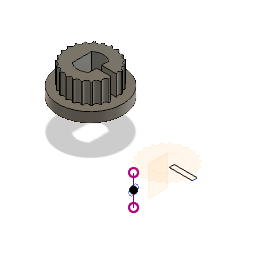
fully-gear v4 (Autodesk Fusion 360 design; units mm, degrees)
Autodesk Fusion 360 part; units mm, degrees
sketch "Sketch1" plane through (0, 0, 0) normal (0, 1, 0) x (1, 0, 0)
  arc A0 (-0.5173, 4.9732) -> (0.5937, 4.9646) centre (0.04, 5.1956) ccw
  arc A1 (-1.8399, 4.6492) -> (-0.7677, 4.9407) centre (-1.3633, 5.0137) ccw
  arc A2 (-3.026, 3.9804) -> (-2.0722, 4.5504) centre (-2.6654, 4.46) ccw
  arc A3 (-3.9877, 3.0164) -> (-3.2231, 3.8225) centre (-3.7698, 3.5755) ccw
  arc A4 (-4.6536, 1.8287) -> (-4.1349, 2.8112) centre (-4.5947, 2.4258) ccw
  arc A5 (-4.9744, 0.5053) -> (-4.74, 1.5914) centre (-5.0788, 1.0962) ccw
  arc A6 (-4.9263, -0.8555) -> (-4.9936, 0.2535) centre (-5.1862, -0.3147) ccw
  arc A7 (-4.5128, -2.1528) -> (-4.8768, -1.1031) centre (-4.909, -1.7022) ccw
  arc A8 (-3.7646, -3.2905) -> (-4.3983, -2.3779) centre (-4.2677, -2.9635) ccw
  arc A9 (-2.7372, -4.1842) -> (-3.5937, -3.4764) centre (-3.3099, -4.005) ccw
  arc A10 (-1.5068, -4.7675) -> (-2.5225, -4.3171) centre (-2.1066, -4.7495) ccw
  arc A11 (-0.1647, -4.9973) -> (-1.2642, -4.8375) centre (-0.7471, -5.1417) ccw
  arc A12 (1.1897, -4.8564) -> (0.0878, -4.9992) centre (0.6679, -5.1526) ccw
  arc A13 (2.4558, -4.3554) -> (1.4333, -4.7902) centre (2.0333, -4.7814) ccw
  arc A14 (3.5398, -3.5313) -> (2.6726, -4.2258) centre (3.2479, -4.0555) ccw
  arc A15 (4.3612, -2.4453) -> (3.7136, -3.3481) centre (4.2216, -3.0288) ccw
  arc A16 (4.8593, -1.178) -> (4.4791, -2.222) centre (4.8822, -1.7775) ccw
  arc A17 (4.9969, 0.1767) -> (4.9125, -0.9311) centre (5.1807, -0.3944) ccw
  arc A18 (4.7639, 1.5183) -> (4.9816, 0.4288) centre (5.095, 1.0179) ccw
  arc A19 (4.1776, 2.7473) -> (4.6812, 1.7569) centre (4.6315, 2.3548) ccw
  arc A20 (3.2815, 3.7725) -> (4.0336, 2.9547) centre (3.8244, 3.5171) ccw
  arc A21 (2.142, 4.518) -> (3.0868, 3.9334) centre (2.7337, 4.4184) ccw
  arc A22 (0.8436, 4.9283) -> (1.9112, 4.6203) centre (1.4402, 4.9921) ccw
  arc A23 (4.1776, 2.7473) -> (4.0336, 2.9547) centre (0, 0) ccw
  arc A24 (4.7639, 1.5183) -> (4.6812, 1.7569) centre (0, 0) ccw
  arc A25 (3.2815, 3.7725) -> (3.0868, 3.9334) centre (0, 0) ccw
  arc A26 (2.142, 4.518) -> (1.9112, 4.6203) centre (0, 0) ccw
  arc A27 (0.8436, 4.9283) -> (0.5937, 4.9646) centre (0, 0) ccw
  arc A28 (-0.5173, 4.9732) -> (-0.7677, 4.9407) centre (0, 0) ccw
  arc A29 (-1.8399, 4.6492) -> (-2.0722, 4.5504) centre (0, 0) ccw
  arc A30 (-3.026, 3.9804) -> (-3.2231, 3.8225) centre (0, 0) ccw
  arc A31 (-3.9877, 3.0164) -> (-4.1349, 2.8112) centre (0, 0) ccw
  arc A32 (-4.6536, 1.8287) -> (-4.74, 1.5914) centre (0, 0) ccw
  arc A33 (-4.9744, 0.5053) -> (-4.9936, 0.2535) centre (0, 0) ccw
  arc A34 (-4.9263, -0.8555) -> (-4.8768, -1.1031) centre (0, 0) ccw
  arc A35 (-4.5128, -2.1528) -> (-4.3983, -2.3779) centre (0, 0) ccw
  arc A36 (-3.7646, -3.2905) -> (-3.5937, -3.4764) centre (0, 0) ccw
  arc A37 (-2.7372, -4.1842) -> (-2.5225, -4.3171) centre (0, 0) ccw
  arc A38 (-1.5068, -4.7675) -> (-1.2642, -4.8375) centre (0, 0) ccw
  arc A39 (-0.1647, -4.9973) -> (0.0878, -4.9992) centre (0, 0) ccw
  arc A40 (1.1897, -4.8564) -> (1.4333, -4.7902) centre (0, 0) ccw
  arc A41 (2.4558, -4.3554) -> (2.6726, -4.2258) centre (0, 0) ccw
  arc A42 (3.5398, -3.5313) -> (3.7136, -3.3481) centre (0, 0) ccw
  arc A43 (4.3612, -2.4453) -> (4.4791, -2.222) centre (0, 0) ccw
  arc A44 (4.8593, -1.178) -> (4.9125, -0.9311) centre (0, 0) ccw
  arc A45 (4.9969, 0.1767) -> (4.9816, 0.4288) centre (0, 0) ccw
  dimension "d1" = 10
  dimension "d2" = 0.6
  dimension "d4" = 360
  measures "d1" diameter of A25
  measures "d2" radius of A0
sketch "Sketch2" plane through (0.0017, 0, 0.0141) normal (0, 1, 0) x (1, 0, 0)
  line L0 (1.7, 1.9007) -> (1.7, -1.9672)
  line L1 (-1.7017, -1.9658) -> (-1.7017, 1.8992)
  arc A0 (-1.7017, -1.9658) -> (1.7, -1.9672) centre (0, 0) ccw
  arc A1 (1.7, 1.9007) -> (-1.7017, 1.8992) centre (0, 0) ccw
  dimension "d5" = 5.2
  dimension "d7" = 1.7
  dimension "d12" = 1.7
  measures "d5" diameter of A0
  measures "d7" distance of L1
  measures "d12" distance of L0 A0.centre
extrude "Extrude1" add sketch "Sketch1" along normal blind 6.1 makes body 1
extrude "Extrude2" cut sketch "Sketch2" along normal blind 12.5 bodies 1
sketch "Sketch3" plane through (-1.7, 0, 0) normal (1, 0, 0) x (0, 0, -1)
  line L0 (1.885, 6.1) -> (-1.9799, 6.1)
  line L1 (-1.9799, 6.1) -> (-1.9799, 0)
  line L2 (-1.9799, 0) -> (1.885, 0)
  line L3 (1.885, 0) -> (1.885, 6.1)
  circle A0 centre (-4.9992, 3.05) radius 0.947
  line L4 (-4.9992, 0) -> (-4.9992, 6.1)
sketch "Sketch4" plane through (0, 6.1, 0) normal (0, 1, 0) x (-1, 0, 0)
  line L0 (1.7, 1.9799) -> (1.7, -1.885)
  arc A0 (-1.7017, -1.8865) -> (1.7, -1.885) centre (-0.0017, 0.0141) ccw
  line L1 (-1.7017, -1.8865) -> (-1.7017, 1.9814)
  arc A1 (1.7, 1.9799) -> (-1.7017, 1.9814) centre (-0.0017, 0.0141) ccw
  arc A2 (-4.8593, 1.178) -> (-4.9125, 0.9311) centre (0, 0) ccw
  arc A3 (-4.9969, -0.1767) -> (-4.9125, 0.9311) centre (-5.1807, 0.3944) ccw
  arc A4 (-4.9969, -0.1767) -> (-4.9816, -0.4288) centre (0, 0) ccw
  arc A5 (-4.7639, -1.5183) -> (-4.9816, -0.4288) centre (-5.095, -1.0179) ccw
  arc A6 (-4.7639, -1.5183) -> (-4.6812, -1.7569) centre (0, 0) ccw
  arc A7 (-4.1776, -2.7473) -> (-4.6812, -1.7569) centre (-4.6315, -2.3548) ccw
  arc A8 (-4.1776, -2.7473) -> (-4.0336, -2.9547) centre (0, 0) ccw
  arc A9 (-3.2815, -3.7725) -> (-4.0336, -2.9547) centre (-3.8244, -3.5171) ccw
  arc A10 (-3.2815, -3.7725) -> (-3.0868, -3.9334) centre (0, 0) ccw
  arc A11 (-2.142, -4.518) -> (-3.0868, -3.9334) centre (-2.7337, -4.4184) ccw
  arc A12 (-2.142, -4.518) -> (-1.9112, -4.6203) centre (0, 0) ccw
  arc A13 (-0.8436, -4.9283) -> (-1.9112, -4.6203) centre (-1.4402, -4.9921) ccw
  arc A14 (-0.8436, -4.9283) -> (-0.5937, -4.9646) centre (0, 0) ccw
  arc A15 (0.5173, -4.9732) -> (-0.5937, -4.9646) centre (-0.04, -5.1956) ccw
  arc A16 (0.5173, -4.9732) -> (0.7677, -4.9407) centre (0, 0) ccw
  arc A17 (1.8399, -4.6492) -> (0.7677, -4.9407) centre (1.3633, -5.0137) ccw
  arc A18 (1.8399, -4.6492) -> (2.0722, -4.5504) centre (0, 0) ccw
  arc A19 (3.026, -3.9804) -> (2.0722, -4.5504) centre (2.6654, -4.46) ccw
  arc A20 (3.026, -3.9804) -> (3.2231, -3.8225) centre (0, 0) ccw
  arc A21 (3.9877, -3.0164) -> (3.2231, -3.8225) centre (3.7698, -3.5755) ccw
  arc A22 (3.9877, -3.0164) -> (4.1349, -2.8112) centre (0, 0) ccw
  arc A23 (4.6536, -1.8287) -> (4.1349, -2.8112) centre (4.5947, -2.4258) ccw
  arc A24 (4.6536, -1.8287) -> (4.74, -1.5914) centre (0, 0) ccw
  arc A25 (4.9744, -0.5053) -> (4.74, -1.5914) centre (5.0788, -1.0962) ccw
  arc A26 (4.9744, -0.5053) -> (4.9936, -0.2535) centre (0, 0) ccw
  arc A27 (4.9263, 0.8555) -> (4.9936, -0.2535) centre (5.1862, 0.3147) ccw
  arc A28 (4.9263, 0.8555) -> (4.8768, 1.1031) centre (0, 0) ccw
  arc A29 (4.5128, 2.1528) -> (4.8768, 1.1031) centre (4.909, 1.7022) ccw
  arc A30 (4.5128, 2.1528) -> (4.3983, 2.3779) centre (0, 0) ccw
  arc A31 (3.7646, 3.2905) -> (4.3983, 2.3779) centre (4.2677, 2.9635) ccw
  arc A32 (3.7646, 3.2905) -> (3.5937, 3.4764) centre (0, 0) ccw
  arc A33 (2.7372, 4.1842) -> (3.5937, 3.4764) centre (3.3099, 4.005) ccw
  arc A34 (2.7372, 4.1842) -> (2.5225, 4.3171) centre (0, 0) ccw
  arc A35 (1.5068, 4.7675) -> (2.5225, 4.3171) centre (2.1066, 4.7495) ccw
  arc A36 (1.5068, 4.7675) -> (1.2642, 4.8375) centre (0, 0) ccw
  arc A37 (0.1647, 4.9973) -> (1.2642, 4.8375) centre (0.7471, 5.1417) ccw
  arc A38 (0.1647, 4.9973) -> (-0.0878, 4.9992) centre (0, 0) ccw
  arc A39 (-1.1897, 4.8564) -> (-0.0878, 4.9992) centre (-0.6679, 5.1526) ccw
  arc A40 (-1.1897, 4.8564) -> (-1.4333, 4.7902) centre (0, 0) ccw
  arc A41 (-2.4558, 4.3554) -> (-1.4333, 4.7902) centre (-2.0333, 4.7814) ccw
  arc A42 (-2.4558, 4.3554) -> (-2.6726, 4.2258) centre (0, 0) ccw
  arc A43 (-3.5398, 3.5313) -> (-2.6726, 4.2258) centre (-3.2479, 4.0555) ccw
  arc A44 (-3.5398, 3.5313) -> (-3.7136, 3.3481) centre (0, 0) ccw
  arc A45 (-4.3612, 2.4453) -> (-3.7136, 3.3481) centre (-4.2216, 3.0288) ccw
  arc A46 (-4.3612, 2.4453) -> (-4.4791, 2.222) centre (0, 0) ccw
  arc A47 (-4.8593, 1.178) -> (-4.4791, 2.222) centre (-4.8822, 1.7775) ccw
ref_plane "WorkPlane2" through (0, 3.1, 0) normal (0, 1, 0) x (-1, 0, 0)
sketch "Sketch6" plane through (0, 6.1, 0) normal (0, 1, 0) x (-1, 0, 0)
  line L0 (1.7, 1.9799) -> (1.7, -1.885)
  arc A0 (-1.7017, -1.8865) -> (1.7, -1.885) centre (-0.0017, 0.0141) ccw
  line L1 (-1.7017, -1.8865) -> (-1.7017, 1.9814)
  arc A1 (1.7, 1.9799) -> (-1.7017, 1.9814) centre (-0.0017, 0.0141) ccw
  arc A2 (-4.8593, 1.178) -> (-4.9125, 0.9311) centre (0, 0) ccw
  arc A3 (-4.9969, -0.1767) -> (-4.9125, 0.9311) centre (-5.1807, 0.3944) ccw
  arc A4 (-4.9969, -0.1767) -> (-4.9816, -0.4288) centre (0, 0) ccw
  arc A5 (-4.7639, -1.5183) -> (-4.9816, -0.4288) centre (-5.095, -1.0179) ccw
  arc A6 (-4.7639, -1.5183) -> (-4.6812, -1.7569) centre (0, 0) ccw
  arc A7 (-4.1776, -2.7473) -> (-4.6812, -1.7569) centre (-4.6315, -2.3548) ccw
  arc A8 (-4.1776, -2.7473) -> (-4.0336, -2.9547) centre (0, 0) ccw
  arc A9 (-3.2815, -3.7725) -> (-4.0336, -2.9547) centre (-3.8244, -3.5171) ccw
  arc A10 (-3.2815, -3.7725) -> (-3.0868, -3.9334) centre (0, 0) ccw
  arc A11 (-2.142, -4.518) -> (-3.0868, -3.9334) centre (-2.7337, -4.4184) ccw
  arc A12 (-2.142, -4.518) -> (-1.9112, -4.6203) centre (0, 0) ccw
  arc A13 (-0.8436, -4.9283) -> (-1.9112, -4.6203) centre (-1.4402, -4.9921) ccw
  arc A14 (-0.8436, -4.9283) -> (-0.5937, -4.9646) centre (0, 0) ccw
  arc A15 (0.5173, -4.9732) -> (-0.5937, -4.9646) centre (-0.04, -5.1956) ccw
  arc A16 (0.5173, -4.9732) -> (0.7677, -4.9407) centre (0, 0) ccw
  arc A17 (1.8399, -4.6492) -> (0.7677, -4.9407) centre (1.3633, -5.0137) ccw
  arc A18 (1.8399, -4.6492) -> (2.0722, -4.5504) centre (0, 0) ccw
  arc A19 (3.026, -3.9804) -> (2.0722, -4.5504) centre (2.6654, -4.46) ccw
  arc A20 (3.026, -3.9804) -> (3.2231, -3.8225) centre (0, 0) ccw
  arc A21 (3.9877, -3.0164) -> (3.2231, -3.8225) centre (3.7698, -3.5755) ccw
  arc A22 (3.9877, -3.0164) -> (4.1349, -2.8112) centre (0, 0) ccw
  arc A23 (4.6536, -1.8287) -> (4.1349, -2.8112) centre (4.5947, -2.4258) ccw
  arc A24 (4.6536, -1.8287) -> (4.74, -1.5914) centre (0, 0) ccw
  arc A25 (4.9744, -0.5053) -> (4.74, -1.5914) centre (5.0788, -1.0962) ccw
  arc A26 (4.9744, -0.5053) -> (4.9936, -0.2535) centre (0, 0) ccw
  arc A27 (4.9263, 0.8555) -> (4.9936, -0.2535) centre (5.1862, 0.3147) ccw
  arc A28 (4.9263, 0.8555) -> (4.8768, 1.1031) centre (0, 0) ccw
  arc A29 (4.5128, 2.1528) -> (4.8768, 1.1031) centre (4.909, 1.7022) ccw
  arc A30 (4.5128, 2.1528) -> (4.3983, 2.3779) centre (0, 0) ccw
  arc A31 (3.7646, 3.2905) -> (4.3983, 2.3779) centre (4.2677, 2.9635) ccw
  arc A32 (3.7646, 3.2905) -> (3.5937, 3.4764) centre (0, 0) ccw
  arc A33 (2.7372, 4.1842) -> (3.5937, 3.4764) centre (3.3099, 4.005) ccw
  arc A34 (2.7372, 4.1842) -> (2.5225, 4.3171) centre (0, 0) ccw
  arc A35 (1.5068, 4.7675) -> (2.5225, 4.3171) centre (2.1066, 4.7495) ccw
  arc A36 (1.5068, 4.7675) -> (1.2642, 4.8375) centre (0, 0) ccw
  arc A37 (0.1647, 4.9973) -> (1.2642, 4.8375) centre (0.7471, 5.1417) ccw
  arc A38 (0.1647, 4.9973) -> (-0.0878, 4.9992) centre (0, 0) ccw
  arc A39 (-1.1897, 4.8564) -> (-0.0878, 4.9992) centre (-0.6679, 5.1526) ccw
  arc A40 (-1.1897, 4.8564) -> (-1.4333, 4.7902) centre (0, 0) ccw
  arc A41 (-2.4558, 4.3554) -> (-1.4333, 4.7902) centre (-2.0333, 4.7814) ccw
  arc A42 (-2.4558, 4.3554) -> (-2.6726, 4.2258) centre (0, 0) ccw
  arc A43 (-3.5398, 3.5313) -> (-2.6726, 4.2258) centre (-3.2479, 4.0555) ccw
  arc A44 (-3.5398, 3.5313) -> (-3.7136, 3.3481) centre (0, 0) ccw
  arc A45 (-4.3612, 2.4453) -> (-3.7136, 3.3481) centre (-4.2216, 3.0288) ccw
  arc A46 (-4.3612, 2.4453) -> (-4.4791, 2.222) centre (0, 0) ccw
  arc A47 (-4.8593, 1.178) -> (-4.4791, 2.222) centre (-4.8822, 1.7775) ccw
  circle A48 centre (0, 0) radius 6
  dimension "d25" = 12
  measures "d25" diameter of A48
sketch "Sketch8" plane through (0, 6.1, 0) normal (0, 1, 0) x (-1, 0, 0)
  line L0 (1.7, 1.9799) -> (1.7, -1.885)
  arc A0 (-1.7017, -1.8865) -> (1.7, -1.885) centre (-0.0017, 0.0141) ccw
  line L1 (-1.7017, -1.8865) -> (-1.7017, 1.9814)
  arc A1 (1.7, 1.9799) -> (-1.7017, 1.9814) centre (-0.0017, 0.0141) ccw
  arc A2 (-4.8593, 1.178) -> (-4.9125, 0.9311) centre (0, 0) ccw
  arc A3 (-4.9969, -0.1767) -> (-4.9125, 0.9311) centre (-5.1807, 0.3944) ccw
  arc A4 (-4.9969, -0.1767) -> (-4.9816, -0.4288) centre (0, 0) ccw
  arc A5 (-4.7639, -1.5183) -> (-4.9816, -0.4288) centre (-5.095, -1.0179) ccw
  arc A6 (-4.7639, -1.5183) -> (-4.6812, -1.7569) centre (0, 0) ccw
  arc A7 (-4.1776, -2.7473) -> (-4.6812, -1.7569) centre (-4.6315, -2.3548) ccw
  arc A8 (-4.1776, -2.7473) -> (-4.0336, -2.9547) centre (0, 0) ccw
  arc A9 (-3.2815, -3.7725) -> (-4.0336, -2.9547) centre (-3.8244, -3.5171) ccw
  arc A10 (-3.2815, -3.7725) -> (-3.0868, -3.9334) centre (0, 0) ccw
  arc A11 (-2.142, -4.518) -> (-3.0868, -3.9334) centre (-2.7337, -4.4184) ccw
  arc A12 (-2.142, -4.518) -> (-1.9112, -4.6203) centre (0, 0) ccw
  arc A13 (-0.8436, -4.9283) -> (-1.9112, -4.6203) centre (-1.4402, -4.9921) ccw
  arc A14 (-0.8436, -4.9283) -> (-0.5937, -4.9646) centre (0, 0) ccw
  arc A15 (0.5173, -4.9732) -> (-0.5937, -4.9646) centre (-0.04, -5.1956) ccw
  arc A16 (0.5173, -4.9732) -> (0.7677, -4.9407) centre (0, 0) ccw
  arc A17 (1.8399, -4.6492) -> (0.7677, -4.9407) centre (1.3633, -5.0137) ccw
  arc A18 (1.8399, -4.6492) -> (2.0722, -4.5504) centre (0, 0) ccw
  arc A19 (3.026, -3.9804) -> (2.0722, -4.5504) centre (2.6654, -4.46) ccw
  arc A20 (3.026, -3.9804) -> (3.2231, -3.8225) centre (0, 0) ccw
  arc A21 (3.9877, -3.0164) -> (3.2231, -3.8225) centre (3.7698, -3.5755) ccw
  arc A22 (3.9877, -3.0164) -> (4.1349, -2.8112) centre (0, 0) ccw
  arc A23 (4.6536, -1.8287) -> (4.1349, -2.8112) centre (4.5947, -2.4258) ccw
  arc A24 (4.6536, -1.8287) -> (4.74, -1.5914) centre (0, 0) ccw
  arc A25 (4.9744, -0.5053) -> (4.74, -1.5914) centre (5.0788, -1.0962) ccw
  arc A26 (4.9744, -0.5053) -> (4.9936, -0.2535) centre (0, 0) ccw
  arc A27 (4.9263, 0.8555) -> (4.9936, -0.2535) centre (5.1862, 0.3147) ccw
  arc A28 (4.9263, 0.8555) -> (4.8768, 1.1031) centre (0, 0) ccw
  arc A29 (4.5128, 2.1528) -> (4.8768, 1.1031) centre (4.909, 1.7022) ccw
  arc A30 (4.5128, 2.1528) -> (4.3983, 2.3779) centre (0, 0) ccw
  arc A31 (3.7646, 3.2905) -> (4.3983, 2.3779) centre (4.2677, 2.9635) ccw
  arc A32 (3.7646, 3.2905) -> (3.5937, 3.4764) centre (0, 0) ccw
  arc A33 (2.7372, 4.1842) -> (3.5937, 3.4764) centre (3.3099, 4.005) ccw
  arc A34 (2.7372, 4.1842) -> (2.5225, 4.3171) centre (0, 0) ccw
  arc A35 (1.5068, 4.7675) -> (2.5225, 4.3171) centre (2.1066, 4.7495) ccw
  arc A36 (1.5068, 4.7675) -> (1.2642, 4.8375) centre (0, 0) ccw
  arc A37 (0.1647, 4.9973) -> (1.2642, 4.8375) centre (0.7471, 5.1417) ccw
  arc A38 (0.1647, 4.9973) -> (-0.0878, 4.9992) centre (0, 0) ccw
  arc A39 (-1.1897, 4.8564) -> (-0.0878, 4.9992) centre (-0.6679, 5.1526) ccw
  arc A40 (-1.1897, 4.8564) -> (-1.4333, 4.7902) centre (0, 0) ccw
  arc A41 (-2.4558, 4.3554) -> (-1.4333, 4.7902) centre (-2.0333, 4.7814) ccw
  arc A42 (-2.4558, 4.3554) -> (-2.6726, 4.2258) centre (0, 0) ccw
  arc A43 (-3.5398, 3.5313) -> (-2.6726, 4.2258) centre (-3.2479, 4.0555) ccw
  arc A44 (-3.5398, 3.5313) -> (-3.7136, 3.3481) centre (0, 0) ccw
  arc A45 (-4.3612, 2.4453) -> (-3.7136, 3.3481) centre (-4.2216, 3.0288) ccw
  arc A46 (-4.3612, 2.4453) -> (-4.4791, 2.222) centre (0, 0) ccw
  arc A47 (-4.8593, 1.178) -> (-4.4791, 2.222) centre (-4.8822, 1.7775) ccw
  line L2 (-1, -0.5) -> (-5.6673, -0.5)
  line L3 (-5.6673, -0.5) -> (-5.6673, 0.5)
  line L4 (-5.6673, 0.5) -> (-1, 0.5)
  line L5 (-1, 0.5) -> (-1, -0.5)
  dimension "d31" = 1
  dimension "d32" = 1
  dimension "d33" = 0.5
extrude "Extrude5" cut sketch "Sketch8" against normal blind 12.5 contours L1 L2 L4 L5 | L1 A3 A4 A5 L2 L4 bodies 1
sketch "Sketch9" plane through (0, 6.1, 0) normal (0, 1, 0) x (-1, 0, 0)
  line L0 (-1.7017, -0.5) -> (-4.7922, -0.5)
  arc A0 (-4.7639, -1.5183) -> (-4.7922, -0.5) centre (-5.095, -1.0179) ccw
  arc A1 (-4.7639, -1.5183) -> (-4.6812, -1.7569) centre (0, 0) ccw
  arc A2 (-4.1776, -2.7473) -> (-4.6812, -1.7569) centre (-4.6315, -2.3548) ccw
  arc A3 (-4.1776, -2.7473) -> (-4.0336, -2.9547) centre (0, 0) ccw
  arc A4 (-3.2815, -3.7725) -> (-4.0336, -2.9547) centre (-3.8244, -3.5171) ccw
  arc A5 (-3.2815, -3.7725) -> (-3.0868, -3.9334) centre (0, 0) ccw
  arc A6 (-2.142, -4.518) -> (-3.0868, -3.9334) centre (-2.7337, -4.4184) ccw
  arc A7 (-2.142, -4.518) -> (-1.9112, -4.6203) centre (0, 0) ccw
  arc A8 (-0.8436, -4.9283) -> (-1.9112, -4.6203) centre (-1.4402, -4.9921) ccw
  arc A9 (-0.8436, -4.9283) -> (-0.5937, -4.9646) centre (0, 0) ccw
  arc A10 (0.5173, -4.9732) -> (-0.5937, -4.9646) centre (-0.04, -5.1956) ccw
  arc A11 (0.5173, -4.9732) -> (0.7677, -4.9407) centre (0, 0) ccw
  arc A12 (1.8399, -4.6492) -> (0.7677, -4.9407) centre (1.3633, -5.0137) ccw
  arc A13 (1.8399, -4.6492) -> (2.0722, -4.5504) centre (0, 0) ccw
  arc A14 (3.026, -3.9804) -> (2.0722, -4.5504) centre (2.6654, -4.46) ccw
  arc A15 (3.026, -3.9804) -> (3.2231, -3.8225) centre (0, 0) ccw
  arc A16 (3.9877, -3.0164) -> (3.2231, -3.8225) centre (3.7698, -3.5755) ccw
  arc A17 (3.9877, -3.0164) -> (4.1349, -2.8112) centre (0, 0) ccw
  arc A18 (4.6536, -1.8287) -> (4.1349, -2.8112) centre (4.5947, -2.4258) ccw
  arc A19 (4.6536, -1.8287) -> (4.74, -1.5914) centre (0, 0) ccw
  arc A20 (4.9744, -0.5053) -> (4.74, -1.5914) centre (5.0788, -1.0962) ccw
  arc A21 (4.9744, -0.5053) -> (4.9936, -0.2535) centre (0, 0) ccw
  arc A22 (4.9263, 0.8555) -> (4.9936, -0.2535) centre (5.1862, 0.3147) ccw
  arc A23 (4.9263, 0.8555) -> (4.8768, 1.1031) centre (0, 0) ccw
  arc A24 (4.5128, 2.1528) -> (4.8768, 1.1031) centre (4.909, 1.7022) ccw
  arc A25 (4.5128, 2.1528) -> (4.3983, 2.3779) centre (0, 0) ccw
  arc A26 (3.7646, 3.2905) -> (4.3983, 2.3779) centre (4.2677, 2.9635) ccw
  arc A27 (3.7646, 3.2905) -> (3.5937, 3.4764) centre (0, 0) ccw
  arc A28 (2.7372, 4.1842) -> (3.5937, 3.4764) centre (3.3099, 4.005) ccw
  arc A29 (2.7372, 4.1842) -> (2.5225, 4.3171) centre (0, 0) ccw
  arc A30 (1.5068, 4.7675) -> (2.5225, 4.3171) centre (2.1066, 4.7495) ccw
  arc A31 (1.5068, 4.7675) -> (1.2642, 4.8375) centre (0, 0) ccw
  arc A32 (0.1647, 4.9973) -> (1.2642, 4.8375) centre (0.7471, 5.1417) ccw
  arc A33 (0.1647, 4.9973) -> (-0.0878, 4.9992) centre (0, 0) ccw
  arc A34 (-1.1897, 4.8564) -> (-0.0878, 4.9992) centre (-0.6679, 5.1526) ccw
  arc A35 (-1.1897, 4.8564) -> (-1.4333, 4.7902) centre (0, 0) ccw
  arc A36 (-2.4558, 4.3554) -> (-1.4333, 4.7902) centre (-2.0333, 4.7814) ccw
  arc A37 (-2.4558, 4.3554) -> (-2.6726, 4.2258) centre (0, 0) ccw
  arc A38 (-3.5398, 3.5313) -> (-2.6726, 4.2258) centre (-3.2479, 4.0555) ccw
  arc A39 (-3.5398, 3.5313) -> (-3.7136, 3.3481) centre (0, 0) ccw
  arc A40 (-4.3612, 2.4453) -> (-3.7136, 3.3481) centre (-4.2216, 3.0288) ccw
  arc A41 (-4.3612, 2.4453) -> (-4.4791, 2.222) centre (0, 0) ccw
  arc A42 (-4.8593, 1.178) -> (-4.4791, 2.222) centre (-4.8822, 1.7775) ccw
  arc A43 (-4.8593, 1.178) -> (-4.9125, 0.9311) centre (0, 0) ccw
  arc A44 (-4.5901, 0.5) -> (-4.9125, 0.9311) centre (-5.1807, 0.3944) ccw
  line L1 (-4.5901, 0.5) -> (-1.7017, 0.5)
  line L2 (1.7, 1.9799) -> (1.7, -1.885)
  arc A45 (-1.7017, -1.8865) -> (1.7, -1.885) centre (-0.0017, 0.0141) ccw
  line L3 (-1.7017, 0.5) -> (-1.7017, 1.9814)
  arc A46 (1.7, 1.9799) -> (-1.7017, 1.9814) centre (-0.0017, 0.0141) ccw
  circle A47 centre (19.267, -3.892) radius 6.5
  line L4 (-1.7017, -1.8865) -> (-1.7017, -0.5)
  dimension "d37" = 13
  measures "d37" diameter of A47
extrude "Extrude6" add sketch "Sketch9" along normal blind 2 separate body contours A47 makes body 2
move_body "Move1" bodies 1 to x (1, 0, 0) y (0, 1, 0) z (0, 0, 1) at (-19.2687, 6.1, -3.9062)
combine "Combine1" operation add target body 1 tool bodies 2
sketch "Sketch10" plane through (0, 6.1, 0) normal (0, -1, 0) x (1, 0, 0)
  circle A0 centre (-19.267, -3.892) radius 6.5
extrude "Extrude7" add sketch "Sketch8" sketch "Sketch4" against normal blind 15 separate body contours L0 A0 L1 A1 L2 L4 L5 of sketch 2 contours L0 A0 L1 A1 makes body 3
move_body "Move2" bodies 3 to x (1, 0, 0) y (0, 1, 0) z (0, 0, 1) at (-19.267, 0, -3.892)
move_body "Move3" bodies 3 to x (1, 0, 0) y (0, 1, 0) z (0, 0, 1) at (0, 8, 0)
combine "Combine2" operation cut target body 1 tool bodies 3
